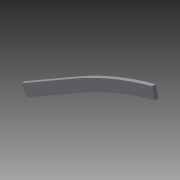
# Autodesk Inventor part: nd-15
Saved by Autodesk Inventor 2015 (Build 190159000, 159)
## iProperties
Created: 2014-07-02
Part Number: nd-15
Material: Generic
Document SubType Name: Modeling
Designer: peter
Density: 1 g/cm^3
Appearance: Default
Author: peter
Autodesk Inventor part; units mm, degrees
ref_plane "YZ Plane" through (0, 0, 0) normal (1, 0, 0) x (0, 1, 0)
ref_plane "XZ Plane" through (0, 0, 0) normal (0, 1, 0) x (-1, 0, 0)
ref_plane "XY Plane" through (0, 0, 0) normal (0, 0, 1) x (1, 0, 0)
sketch "Sketch1" plane through (0, 0, 0) normal (0, 0, 1) x (1, 0, 0)
  arc A0 (674.48, 374.6273) -> (275.278, 208.3151) centre (1116.653, -1248.9892) ccw
  line L0 (275.278, 208.3151) -> (0.0426, 49.4078)
  line L1 (0.0426, 49.4078) -> (28.6176, -0.0855)
  line L2 (28.6176, -0.0855) -> (303.853, 158.8217)
  arc A1 (695.9168, 321.2198) -> (303.853, 158.8217) centre (1116.653, -1248.9892) ccw
  line L3 (695.9168, 321.2198) -> (681.1253, 376.4225)
  arc A2 (681.1253, 376.4225) -> (275.278, 208.3151) centre (1116.653, -1248.9892) ccw
  line L4 (275.278, 208.3151) -> (0.0426, 49.4078)
  point P0 (0, 0)
  constraints: 10 end point, 7 point on circle, 3 centre point
extrude "Extrusion1" add sketch "Sketch1" along normal blind 19.05
body "Solid1"
